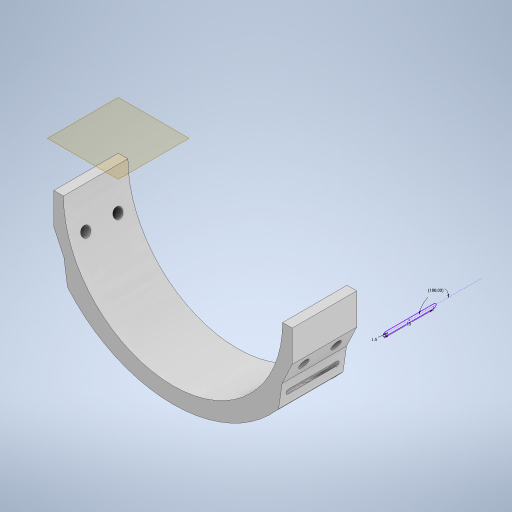
# Autodesk Inventor part: RatMRIPETCTAdapterV3_20mm
Saved by Autodesk Inventor 2023 (Build 270158030, 158C)
## iProperties
Created: 2023-03-23
Part Number: RatMRIPETCTAdapterV3_20mm
Material: Generic
Document SubType Name: Modeling
Designer: sqa4002
Density: 1 g/cm^3
Appearance: Default
Author: sqa4002
Autodesk Inventor part; units mm, degrees
ref_plane "YZ Plane" through (0, 0, 0) normal (1, 0, 0) x (0, 1, 0)
ref_plane "XZ Plane" through (0, 0, 0) normal (0, 1, 0) x (-1, 0, 0)
ref_plane "XY Plane" through (0, 0, 0) normal (0, 0, 1) x (1, 0, 0)
sketch "Sketch1" plane through (0, 0, 0) normal (0, 0, 1) x (1, 0, 0)
  arc A0 (-34, -4) -> (34, -4) centre (0, -4) ccw
  line L0 (-34, -4) -> (-26.1812, -4)
  line L1 (34, -4) -> (26.1812, -4)
  line L2 (-26.1812, -4) -> (-26.1812, -8.6531)
  line L3 (26.1812, -4) -> (26.1812, -8.6531)
  line L4 (-26.1812, -8.6531) -> (-29.5916, -10.258)
  line L5 (26.1812, -8.6531) -> (29.5916, -10.258)
  line L6 (-29.5916, -10.258) -> (-26.4408, -16.9537)
  line L7 (29.5916, -10.258) -> (26.4408, -16.9537)
  line L8 (-26.4408, -16.9537) -> (-23.5453, -15.5911)
  line L9 (26.4408, -16.9537) -> (23.5453, -15.5911)
  line L10 (-23.5453, -15.5911) -> (-20.6171, -21.8136)
  line L11 (23.5453, -15.5911) -> (20.6171, -21.8136)
  line L12 (-20.6171, -21.8136) -> (-20.6171, -23.8136)
  line L13 (20.6171, -21.8136) -> (20.6171, -23.8136)
  arc A1 (-20.6171, -23.8136) -> (-15.6171, -28.8136) centre (-15.6171, -23.8136) ccw
  arc A2 (15.6171, -28.8136) -> (20.6171, -23.8136) centre (15.6171, -23.8136) ccw
  line L14 (-15.6171, -28.8136) -> (15.6171, -28.8136)
  line L15 (-34, -4) -> (-31.5, -4) construction
  arc A3 (-32.3883, -28.2843) -> (32.3883, -28.2843) centre (0, 0) ccw
  line L16 (-32.75, -27.8646) -> (-32.3883, -28.2843)
  line L17 (32.75, -27.8646) -> (32.3883, -28.2843)
  circle A4 centre (0, 0) radius 45
  line L18 (-34, -4) -> (-37, -4)
  line L19 (-37, -4) -> (-37, -13.7443)
  line L20 (-37, -13.7443) -> (-33.8483, -20.4416)
  line L21 (-33.8483, -20.4416) -> (-32.75, -27.8646)
  line L22 (34, -4) -> (37, -4)
  line L23 (37, -4) -> (37, -13.7443)
  line L24 (37, -13.7443) -> (33.8491, -20.4399)
  line L25 (33.8491, -20.4399) -> (32.75, -27.8646)
  dimension "d0" = 68
  dimension "d1" = 34
  dimension "d2" = 7.8188
  dimension "d3" = 7.8188
  dimension "d4" = 4.6531
  dimension "d5" = 4.6531
  dimension "d6" = 3.7692
  dimension "d7" = 3.7692
  dimension "d8" = 115.201
  dimension "d9" = 115.201
  dimension "d10" = 7.4
  dimension "d11" = 90
  dimension "d12" = 90
  dimension "d13" = 3.2
  dimension "d14" = 90
  dimension "d15" = 3.2
  dimension "d16" = 90
  dimension "d17" = 6.877
  dimension "d18" = 90
  dimension "d19" = 6.877
  dimension "d20" = 90
  dimension "d21" = 2
  dimension "d22" = 5
  dimension "d23" = 5
  dimension "d24" = 31.2343
  dimension "d28" = 4
  dimension "d29" = 90
  dimension "d30" = 3
  dimension "d32" = 3
  dimension "d33" = 9.7443
  constraints: 52 end point, 8 point on circle, 6 horizontal, 5 centre point, 5 vertical, 2 parallel, 1 coincident, 1 perpendicular, 1 point on line
  measures "d0" distance of L0.start L1.start
  measures "d1" radius of A0
  measures "d2" distance of L0.start L0.end
  measures "d3" distance of L1.start L1.end
  measures "d4" distance of L0.end L2.end
  measures "d5" distance of L1.end L3.end
  measures "d6" distance of L2.end L4.end
  measures "d7" distance of L3.end L5.end
  measures "d8" angle of L4 L2
  measures "d9" angle of L5 L3
  measures "d10" distance of L4.end L6.end
  measures "d11" angle of L6 L4
  measures "d12" angle of L7 L5
  measures "d13" distance of L6.end L8.end
  measures "d14" angle of L8 L6
  measures "d15" distance of L7.end L9.end
  measures "d16" angle of L7 L9
  measures "d17" distance of L8.end L10.end
  measures "d18" angle of L10 L8
  measures "d19" distance of L9.end L11.end
  measures "d20" angle of L11 L9
  measures "d21" distance of L10.end L12.end
  measures "d22" radius of A1
  measures "d23" radius of A2
  measures "d24" distance of L14.start L14.end
  measures "d28" distance of point (0, 0) A0.centre
  measures "d29" diameter of A4
  measures "d30" distance of L0.start L18.end
  measures "d32" distance of L1.start L22.end
  measures "d33" distance of L22.end L23.end
extrude "Extrusion1" add sketch "Sketch1" along normal blind 20 contours A0 L22 L23 L24 L25 L17 A3 L16 L21 L20 L19 L18
sketch "Sketch2" plane through (37, -13.7443, 20) normal (0.9048196, -0.4257951, 0) x (0, 0, -1)
  circle A0 centre (5, -3.3183) radius 1.5
  line L0 (0, -7.4) -> (0, 0) projected
  circle A1 centre (15, -3.3183) radius 1.5
  circle A2 centre (25, -3.3183) radius 1.5
  circle A3 centre (35, -3.3183) radius 1.5
  circle A4 centre (45, -3.3183) radius 1.5
  point P0 (20, -3.3183)
  dimension "d36" = 3
  dimension "d37" = 5
  dimension "d38" = 3
  dimension "d39" = 10
  dimension "d40" = 3
  dimension "d41" = 10
  dimension "d42" = 3
  dimension "d43" = 10
  dimension "d44" = 3
  dimension "d45" = 10
  constraints: 5 centre point
  measures "d36" diameter of A0
  measures "d37" distance from line of L0 A0.centre
  measures "d38" diameter of A1
  measures "d39" distance of A1.centre A0.centre
  measures "d40" diameter of A2
  measures "d41" distance of A2.centre A1.centre
  measures "d42" diameter of A3
  measures "d43" distance of A3.centre A2.centre
  measures "d44" diameter of A4
  measures "d45" distance of A4.centre A3.centre
extrude "Extrusion2" cut sketch "Sketch2" against normal up to surface round surface about axis through (0, -4, 0) along (0, 0, 1) radius 34 far side no
sketch "Sketch3" plane through (-33.8483, -20.4416, 0) normal (-0.9048196, -0.4257951, 0) x (0, 0, 1)
  circle A0 centre (5, 4.0835) radius 1.5
  line L0 (0, 7.4019) -> (0, 0) projected
  circle A1 centre (15, 4.0835) radius 1.5
  circle A2 centre (25, 4.0835) radius 1.5
  circle A3 centre (35, 4.0835) radius 1.5
  circle A4 centre (45, 4.0835) radius 1.5
  point P0 (0, 4.0835)
  dimension "d48" = 3
  dimension "d49" = 5
  dimension "d50" = 3
  dimension "d51" = 10
  dimension "d52" = 3
  dimension "d53" = 10
  dimension "d54" = 3
  dimension "d55" = 10
  dimension "d56" = 3
  dimension "d57" = 10
  constraints: 5 centre point
  measures "d48" diameter of A0
  measures "d49" distance from line of A0.centre L0
  measures "d50" diameter of A1
  measures "d51" distance of A1.centre A0.centre
  measures "d52" diameter of A2
  measures "d53" distance of A2.centre A1.centre
  measures "d54" diameter of A3
  measures "d55" distance of A3.centre A2.centre
  measures "d56" diameter of A4
  measures "d57" distance of A4.centre A3.centre
extrude "Extrusion3" cut sketch "Sketch3" against normal up to surface round surface about axis through (0, -4, 0) along (0, 0, 1) radius 34 far side no
ref_plane "Work Plane1" through (-37, 0, 0) normal (0, 1, 0) x (1, 0, 0)
sketch "Sketch5" plane through (-37, 0, 0) normal (0, 1, 0) x (1, 0, 0)
  circle A0 centre (68.25, -15) radius 1.5
  circle A1 centre (5.75, -15) radius 1.5
  line L0 (65.75, -10) -> (65.75, -20) projected
  line L1 (8.25, -20) -> (8.25, -10) projected
  point P0 (37, 0)
  dimension "d85" = 3
  dimension "d86" = 3
  dimension "d87" = 2.5
  dimension "d88" = 2.5
  constraints: 2 centre point
  measures "d85" diameter of A0
  measures "d86" diameter of A1
  measures "d87" distance from line of L0 A0.centre
  measures "d88" distance from line of L1 A1.centre
extrude "Extrusion5" cut sketch "Sketch5" against normal blind 4
sketch "Sketch6" plane through (33.8491, -20.4399, 20) normal (0.9892194, -0.1464409, 0) x (0, 0, -1)
  line L0 (47.5, -3.2047) -> (32.5, -3.2047) construction
  line L1 (47.5, -2.4547) -> (32.5, -2.4547)
  line L2 (32.5, -3.9547) -> (47.5, -3.9547)
  arc A0 (47.5, -3.9547) -> (47.5, -2.4547) centre (47.5, -3.2047) ccw
  arc A1 (32.5, -2.4547) -> (32.5, -3.9547) centre (32.5, -3.2047) ccw
  line L3 (47.5, -3.2047) -> (62.5, -3.2047) construction
  point P0 (20, 15.2627)
  point P1 (20, 6.3268)
  point P2 (40, -3.2047)
  dimension "d73" = 15
  dimension "d74" = 180
  dimension "d75" = 1.5
  constraints: 10 end point, 4 point on circle, 4 tangent, 2 centre point, 1 collinear, 1 horizontal, 1 midpoint, 1 parallel
  measures "d73" distance of L0.start L0.end
  measures "d74" angle of L0 L3
  measures "d75" diameter of A1
sketch "Sketch7" plane through (-32.75, -27.8646, 0) normal (-0.9892302, -0.1463679, 0) x (0, 0, 1)
  line L0 (2.5, 3.7591) -> (17.5, 3.7591) construction
  line L1 (0, 3.7591) -> (20, 3.7591) projected
  line L2 (2.5, 3.0091) -> (17.5, 3.0091)
  line L3 (17.5, 4.5091) -> (2.5, 4.5091)
  arc A0 (2.5, 4.5091) -> (2.5, 3.0091) centre (2.5, 3.7591) ccw
  arc A1 (17.5, 3.0091) -> (17.5, 4.5091) centre (17.5, 3.7591) ccw
  line L4 (2.5, 3.7591) -> (17.5, 3.7591) construction
  line L5 (0, 7.5038) -> (0, 0) projected
  point P0 (0, 22.771)
  point P1 (10, 3.7591)
  dimension "d77" = 15
  dimension "d78" = 0
  dimension "d79" = 1.5
  dimension "d80" = 2.5
  dimension "d82" = 0
  constraints: 10 end point, 4 point on circle, 4 tangent, 2 centre point, 2 collinear, 1 horizontal, 1 midpoint, 1 parallel
  measures "d77" distance of L0.start L0.end
  measures "d78" distance between parallel lines of L0 L4
  measures "d79" diameter of A1
  measures "d80" distance from line of L5 L0.start
  measures "d82" distance from line of L1 L0.start
sketch "Sketch9" plane through (0, 0, 0) normal (0, 0, -1) x (-1, 0, 0)
  line L0 (-32.75, -27.8646) -> (-33.8491, -20.4399) projected
  line L1 (33.8483, -20.4416) -> (32.75, -27.8646) projected
  line L2 (33.8483, -20.4416) -> (32.75, -27.8646) projected
  arc A0 (-33.3803, -23.6068) -> (33.2992, -24.1531) centre (0.1687, 1.6611) ccw
  point P0 (0, 0)
  dimension "d81" = 42
  constraints: 2 point on circle, 1 centre point, 1 midpoint, 1 point on line
  measures "d81" radius of A0
sketch "Sketch10" plane through (33.8491, -20.4399, 20) normal (0.9892194, -0.1464409, 0) x (0, 0, -1)
  line L0 (20, -3.7517) -> (0, -3.7517) projected
  line L1 (2.5, -3.7517) -> (17.5, -3.7517) construction
  line L2 (2.5, -4.5017) -> (17.5, -4.5017)
  line L3 (17.5, -3.0017) -> (2.5, -3.0017)
  arc A0 (2.5, -3.0017) -> (2.5, -4.5017) centre (2.5, -3.7517) ccw
  arc A1 (17.5, -4.5017) -> (17.5, -3.0017) centre (17.5, -3.7517) ccw
  line L4 (0, -7.5056) -> (0, 0) projected
  point P0 (20, 15.2627)
  point P1 (10, -3.7517)
  dimension "d89" = 15
  dimension "d90" = 1.5
  dimension "d91" = 2.5
  constraints: 8 end point, 4 point on circle, 4 tangent, 2 centre point, 2 point on line, 1 midpoint, 1 parallel
  measures "d89" distance of L1.start L1.end
  measures "d90" diameter of A1
  measures "d91" distance from line of L4 L1.start
sweep "Sweep2" cut profiles "Sketch10" path "Sketch9" keep normal constant yes path curves A0
body "Solid1"
